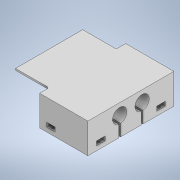
# Autodesk Inventor part: jeffs hair
Saved by Autodesk Inventor 2020 (Build 240168000, 168)
## iProperties
Created: 2023-03-22
Part Number: jeffs hair
Material: Generic
Document SubType Name: Modeling
Designer: user
Density: 1 g/cm^3
Appearance: Default
Author: user
Autodesk Inventor part; units mm, degrees
ref_plane "YZ Plane" through (0, 0, 0) normal (1, 0, 0) x (0, 1, 0)
ref_plane "XZ Plane" through (0, 0, 0) normal (0, 1, 0) x (-1, 0, 0)
sketch "Sketch1" plane through (0, 0, 0) normal (0, 1, 0) x (-1, 0, 0)
  circle A0 centre (7.5, 15) radius 1.25
  circle A1 centre (7.5, 85) radius 1.25
  circle A2 centre (48, 2.5) radius 1.25
  circle A3 centre (48, 97.5) radius 1.25
  line L0 (61, 100) -> (5, 100)
  line L1 (5, 100) -> (5, 0)
  line L2 (5, 0) -> (63, 0)
  line L3 (53, 5) -> (10, 5)
  line L4 (10, 95) -> (61, 95)
  line L5 (61, 89) -> (63, 89)
  line L6 (100, 57.5) -> (100, 89)
  line L7 (100, 89) -> (63, 89)
  line L8 (63, 89) -> (61, 89)
  line L9 (61, 95) -> (10, 95)
  line L10 (10, 95) -> (10, 5)
  line L11 (10, 5) -> (53, 5)
  line L12 (63, 11) -> (100, 11)
  line L13 (100, 11) -> (100, 42.5)
  line L14 (61, 89) -> (61, 100)
  line L15 (61, 11) -> (61, 0)
  line L16 (53, 5) -> (61, 5)
  line L17 (61, 11) -> (63, 11)
  line L18 (100, 57.5) -> (100, 42.5)
  line L19 (95, 89) -> (95, 11)
  dimension "d0" = 5
  dimension "d3" = 100
  dimension "d4" = 95
  dimension "d5" = 5
  dimension "d6" = 5
  dimension "d7" = 5
  constraints: 40 end point, 5 point on line, 4 centre point, 3 perpendicular, 1 parallel, 1 vertical
  measures "d0" distance between parallel lines of L13 L19
  measures "d3" distance of L0.end L1.end
  measures "d4" distance between parallel lines of L6 L1
  measures "d5" distance between parallel lines of L10 L1
  measures "d6" distance between parallel lines of L0 L4
  measures "d7" distance between parallel lines of L2 L3
extrude "Extrusion1" add sketch "Sketch1" along normal blind 2 contours A0 | A1 | A2 | A3 | L14 L4 L10 L3 L16 L15 L2 L1 L0 | L14 L5 L7 L19 L12 L17 L15 L16 L3 L10 L4 | L7 L6 L18 L13 L12 L19
extrude "Extrusion2" add sketch "Sketch1" against normal blind 33 contours L14 L4 L10 L3 L16 L15 L2 L1 L0
sketch "Sketch2" plane through (-5, 2, 100) normal (1, 0, 0) x (0, 0, -1)
  circle A0 centre (37, -13) radius 8.3
  circle A1 centre (63, -13) radius 8.3
  line L0 (100, -35) -> (0, -35) projected
  line L1 (0, -35) -> (0, 0) projected
  line L2 (64, -21.2395) -> (64, -35.2275)
  line L3 (64, -35.2275) -> (62, -35.2275)
  line L4 (62, -35.2275) -> (62, -21.2395)
  line L5 (63.373, -21.2916) -> (64, -35.2275) construction
  line L6 (62.627, -21.2916) -> (62, -35.2275) construction
  line L7 (5, -35) -> (95, -35) projected
  line L8 (50, -35) -> (50, -25.1985)
  line L9 (0, -35) -> (100, -35)
  line L10 (36, -21.2395) -> (36, -35.2275)
  line L11 (36, -35.2275) -> (38, -35.2275)
  line L12 (38, -35.2275) -> (38, -21.2395)
  line L13 (36.627, -21.2916) -> (36, -35.2275) construction
  line L14 (37.373, -21.2916) -> (38, -35.2275) construction
  line L15 (95, -35) -> (5, -35)
  line L16 (46.2725, -3) -> (79.7275, -3)
  line L17 (79.7275, -3) -> (79.7275, -23)
  line L18 (79.7275, -23) -> (46.2725, -23)
  line L19 (46.2725, -23) -> (46.2725, -3)
  line L20 (46.2725, -3) -> (79.7275, -23) construction
  line L21 (79.7275, -3) -> (46.2725, -23) construction
  point P0 (100, -2)
  point P1 (38, -21.2395)
  point P2 (62, -35)
  point P3 (64, -35)
  dimension "d14" = 16.6
  dimension "d15" = 16.6
  dimension "d16" = 26
  dimension "d17" = 22
  dimension "d18" = 37
  dimension "d37" = 2
  dimension "d39" = 20
  constraints: 38 end point, 10 symmetric about line, 4 point on circle, 3 midpoint, 3 parallel, 2 centre point, 1 horizontal, 1 horizontal alignment, 1 perpendicular, 1 vertical
  measures "d14" diameter of A0
  measures "d15" diameter of A1
  measures "d16" distance of A1.centre A0.centre
  measures "d17" distance from line of L0 A0.centre
  measures "d18" distance from line of L1 A0.centre
  measures "d37" distance of L2.end L3.end
  measures "d39" distance of L16.end L17.end
extrude "Extrusion4" cut sketch "Sketch2" against normal blind 10 contours A0 | A0 L12 L0 L10 | L0 L12 L11 L10 | A1 | A1 L2 L18 L4 | L18 L2 L0 L4
sketch "Sketch3" plane through (-10, -33, 5) normal (-1, 0, 0) x (0, 0, 1)
  arc A0 (59, 13.7605) -> (57, 13.7605) centre (58, 22) ccw projected
  arc A1 (33, 13.7605) -> (31, 13.7605) centre (32, 22) ccw projected
  circle A2 centre (58, 22) radius 10
  circle A3 centre (32, 22) radius 10
  line L0 (58, 32) -> (32, 32)
  line L1 (58, 12) -> (32, 12)
  line L2 (39, 36) -> (51, 36)
  line L3 (51, 36) -> (51, 28)
  line L4 (51, 28) -> (39, 28)
  line L5 (39, 28) -> (39, 36)
  line L6 (39, 36) -> (51, 28) construction
  line L7 (51, 36) -> (39, 28) construction
  line L8 (59, 13.7605) -> (59, 0) projected
  line L9 (57, 0) -> (57, 13.7605) projected
  line L10 (33, 13.7605) -> (33, 0) projected
  line L11 (31, 0) -> (31, 13.7605) projected
  point P0 (-5, 33)
  point P1 (45, 32)
  point P2 (39, 32)
  point P3 (51, 32)
  point P4 (33, 12)
  point P5 (57, 12)
  point P6 (59, 12.0501)
  point P7 (51, 29.1414)
  point P8 (39, 29.1414)
  point P9 (31, 12.0501)
  dimension "d21" = 20
  dimension "d22" = 20
  dimension "d24" = 12
  dimension "d25" = 8
  dimension "d38" = 20
  constraints: 16 end point, 4 point on circle, 3 midpoint, 2 centre point, 2 coincident, 2 parallel, 2 tangent, 1 horizontal, 1 perpendicular
  measures "d21" diameter of A2
  measures "d22" diameter of A3
  measures "d24" distance of L3.end L4.end
  measures "d25" distance of L2.end L3.end
  measures "d38" distance between parallel lines of L0 L1
extrude "Extrusion6" add sketch "Sketch3" along normal blind 12 contours A0 L9 A2 L4 L3 L8 | L9 L1 L10 A3 L4 A2 | A3 L10 A1 L11 L5 L4
ref_plane "Work Plane1" through (0, -28, 0) normal (0, -1, 0) x (1, 0, 0)
sketch "Sketch5" plane through (0, -28, 0) normal (0, -1, 0) x (1, 0, 0)
  line L0 (-53, 100) -> (-53, 95) projected
  line L1 (-53, 95) -> (-43, 95) projected
  line L2 (-43, 95) -> (-43, 100) projected
  line L3 (-5, 90) -> (-10, 90) projected
  line L4 (-10, 90) -> (-10, 80) projected
  line L5 (-10, 80) -> (-5, 80) projected
  line L6 (-5, 100) -> (-5, 0) projected
  line L7 (-61, 100) -> (-5, 100) projected
  line L8 (-5, 20) -> (-10, 20) projected
  line L9 (-10, 20) -> (-10, 10) projected
  line L10 (-10, 10) -> (-5, 10) projected
  line L11 (-5, 0) -> (-61, 0) projected
  line L12 (-43, 0) -> (-43, 5) projected
  line L13 (-61, 5) -> (-10, 5) projected
  line L14 (-53, 5) -> (-53, 0) projected
  point P0 (0, 0)
extrude "Extrusion7" cut sketch "Sketch5" against normal blind 5
chamfer "Chamfer1" distance 2 angle 45 2 edges at (-61, 1, 11) (-61, 1, 89)
body "Solid1"
